Autodesk Inventor part; units mm, degrees
(part 2 of 2)
  spline S89 degree 3 poles (1.5423, -31.1895) (1.525, -31.1709) (1.4965, -31.143) (1.4607, -31.1053) (1.4308, -31.0761) (1.3995, -31.0504) (1.3711, -31.0116) (1.3289, -30.9799) (1.2928, -30.9315) (1.2505, -30.9007) (1.2256, -30.8625) (1.198, -30.8522) (1.1849, -30.8167) (1.168, -30.8425) (1.1747, -30.8641) (1.1731, -30.8896) (1.1714, -30.9248) (1.1764, -30.9669) (1.1759, -31.0225) (1.1727, -31.0799) (1.1753, -31.1417) (1.1771, -31.2039) (1.1741, -31.2647) (1.178, -31.3315) (1.1754, -31.4086) (1.1839, -31.5196) (1.1745, -31.7052) (1.1921, -31.8973) (1.1869, -32.1123) (1.2042, -32.2863) (1.2211, -32.4669) (1.2596, -32.6084) (1.3107, -32.7248) (1.3689, -32.8413) (1.4764, -32.9142) (1.5832, -32.9845) (1.7264, -33.001) (1.8989, -33.0107) (2.1172, -33.0071) (2.3634, -33.008) (2.6188, -33.009) (2.8414, -33.0049) (3.021, -33.0145) (3.147, -32.965) (3.2127, -32.8764) (3.2326, -32.7791) (3.2259, -32.6755) (3.2237, -32.54) (3.2294, -32.3531) (3.2274, -32.1408) (3.2295, -31.893) (3.2271, -31.6251) (3.2278, -31.3115) (3.2293, -31.0183) (3.2271, -30.7799) (3.2306, -30.583) (3.2235, -30.4136) (3.2463, -30.2673) (3.1973, -30.187) (3.166, -30.1309) (3.103, -30.0955) (3.0386, -30.0612) (2.9601, -30.073) (2.877, -30.0634) (2.7737, -30.0639) (2.6629, -30.0682) (2.5435, -30.0645) (2.4271, -30.0598) (2.3642, -30.0653) (2.2866, -30.0561) (2.3231, -30.0866) (2.3537, -30.1027) (2.3857, -30.1444) (2.4192, -30.1889) (2.4599, -30.2542) (2.4978, -30.3242) (2.5079, -30.3954) (2.531, -30.4406) (2.5232, -30.4969) (2.5393, -30.5594) (2.5579, -30.6677) (2.575, -30.8097) (2.5711, -30.9741) (2.5797, -31.1302) (2.5874, -31.2728) (2.58, -31.4046) (2.5875, -31.5255) (2.6027, -31.6432) (2.5734, -31.7683) (2.59, -31.8845) (2.58, -31.9915) (2.5914, -32.0945) (2.5752, -32.2046) (2.5838, -32.3311) (2.5772, -32.4642) (2.5844, -32.5873) (2.5862, -32.686) (2.5777, -32.7699) (2.5862, -32.8154) (2.5728, -32.8827) (2.5522, -32.8428) (2.5299, -32.8211) (2.4929, -32.7958) (2.4669, -32.7597) (2.4326, -32.7361) (2.4064, -32.7076) (2.3753, -32.6805) (2.3475, -32.6496) (2.3163, -32.6216) (2.278, -32.5902) (2.241, -32.5379) (2.1844, -32.4937) (2.1417, -32.4408) (2.0971, -32.398) (2.0525, -32.3645) (2.0209, -32.3209) (1.9846, -32.2913) (1.9485, -32.2523) (1.9142, -32.2193) (1.8787, -32.1788) (1.8467, -32.1411) (1.8016, -32.1072) (1.7684, -32.0675) (1.723, -32.0291) (1.6828, -31.984) (1.6372, -31.9322) (1.5828, -31.8839) (1.5289, -31.8255) (1.4793, -31.7809) (1.4402, -31.742) (1.404, -31.7147) (1.3813, -31.6586) (1.3906, -31.5961) (1.3859, -31.5127) (1.383, -31.4312) (1.3904, -31.37) (1.3777, -31.2946) (1.438, -31.3487) (1.4556, -31.3895) (1.502, -31.4233) (1.5317, -31.4575) (1.5733, -31.4877) (1.5975, -31.5313) (1.6422, -31.5628) (1.6696, -31.6065) (1.7072, -31.6387) (1.7424, -31.6701) (1.7691, -31.7071) (1.8115, -31.7333) (1.8439, -31.7668) (1.8879, -31.8131) (1.9321, -31.8595) (1.9919, -31.9083) (2.0296, -31.9505) (2.0756, -32.0014) (2.1275, -32.0517) (2.1924, -32.1161) (2.2393, -32.1725) (2.2909, -32.2076) (2.3009, -32.2368) (2.3275, -32.2565) (2.3371, -32.233) (2.3277, -32.211) (2.3296, -32.1797) (2.3264, -32.1191) (2.324, -31.9699) (2.3296, -31.6728) (2.3328, -31.2678) (2.3082, -30.8815) (2.2811, -30.6221) (2.2452, -30.4786) (2.2139, -30.3874) (2.1709, -30.31) (2.1288, -30.2355) (2.0582, -30.1918) (1.9981, -30.1354) (1.9228, -30.1164) (1.86, -30.0932) (1.7818, -30.0839) (1.7031, -30.0648) (1.6091, -30.0647) (1.5325, -30.0613) (1.4489, -30.0618) (1.2733, -30.0637) (1.0518, -30.061) (0.7618, -30.0612) (0.5648, -30.0623) (0.3839, -30.0834) (0.3326, -30.1673) (0.2783, -30.2266) (0.2949, -30.2944) (0.277, -30.3586) (0.2876, -30.4558) (0.2771, -30.5742) (0.2899, -30.7018) (0.2803, -30.8207) (0.2884, -30.9299) (0.2664, -31.0532) (0.2756, -31.1752) (0.2699, -31.3079) (0.2729, -31.4304) (0.2665, -31.5576) (0.273, -31.6838) (0.2628, -31.8185) (0.2732, -31.9768) (0.2633, -32.1486) (0.2663, -32.3313) (0.2826, -32.4866) (0.2694, -32.6431) (0.275, -32.7606) (0.2877, -32.8635) (0.3306, -32.9345) (0.4067, -32.9774) (0.5101, -33.0018) (0.6141, -32.994) (0.7167, -33.0028) (0.7978, -33.0003) (0.876, -32.9986) (0.9587, -33.0082) (1.0404, -32.9948) (1.1238, -33.0062) (1.1765, -32.9991) (1.2055, -33.008) knots 0 0 0 0 0.003468 0.005439 0.007104 0.009169 0.010945 0.01361 0.016316 0.01908 0.020762 0.022201 0.023332 0.024029 0.025236 0.026466 0.027456 0.030055 0.032225 0.035047 0.037901 0.04066 0.043548 0.046196 0.049786 0.054063 0.061374 0.07511 0.080331 0.090714 0.098946 0.105065 0.110602 0.11639 0.122413 0.128012 0.133614 0.141696 0.151738 0.163348 0.175333 0.186595 0.193786 0.199727 0.204177 0.208239 0.213025 0.218319 0.226749 0.238544 0.247303 0.260584 0.275108 0.290136 0.300597 0.307698 0.31691 0.324166 0.326546 0.3296 0.33273 0.336239 0.339239 0.343233 0.347669 0.353338 0.35828 0.364316 0.367919 0.369623 0.370752 0.372387 0.375037 0.377468 0.380114 0.385513 0.388136 0.389867 0.392271 0.395601 0.398609 0.407302 0.415055 0.421029 0.428641 0.434538 0.439012 0.445186 0.450585 0.456271 0.461021 0.465216 0.470338 0.476105 0.482456 0.48854 0.492838 0.496163 0.499368 0.500865 0.502042 0.503521 0.505691 0.507878 0.509559 0.511315 0.51315 0.515175 0.516985 0.518877 0.521908 0.525642 0.528599 0.531161 0.53407 0.536151 0.538454 0.540425 0.5434 0.544949 0.547785 0.550125 0.552599 0.554817 0.558226 0.560836 0.564232 0.568141 0.571676 0.573323 0.575691 0.577746 0.581215 0.584106 0.589282 0.591694 0.593826 0.595998 0.598671 0.60089 0.603406 0.604911 0.60784 0.610008 0.61224 0.614777 0.616731 0.618675 0.620926 0.623438 0.625015 0.629649 0.632172 0.635539 0.637359 0.641531 0.645414 0.649794 0.651668 0.653476 0.654327 0.654982 0.656131 0.657628 0.659141 0.664473 0.677942 0.699748 0.719713 0.730811 0.735254 0.739899 0.743899 0.747388 0.751337 0.755043 0.758449 0.761723 0.764177 0.769156 0.772731 0.77696 0.779637 0.78414 0.800935 0.809968 0.823451 0.828907 0.832769 0.836469 0.839009 0.841646 0.845448 0.852184 0.857853 0.86287 0.868439 0.87272 0.879862 0.885038 0.890852 0.896577 0.902417 0.908085 0.914984 0.924029 0.931552 0.939919 0.945276 0.95293 0.955988 0.959308 0.96382 0.967488 0.973717 0.977903 0.981537 0.984789 0.988579 0.992845 0.995948 1 1 1 1 construction
  spline S90 degree 3 poles (2.1147, -31.6416) (2.121, -31.666) (2.1095, -31.6932) (2.1202, -31.731) (2.1024, -31.745) (2.0842, -31.7249) (2.0686, -31.6977) (2.0354, -31.6752) (2.0032, -31.6459) (1.9804, -31.6124) (1.9391, -31.5932) (1.9188, -31.5561) (1.8864, -31.5362) (1.8629, -31.5076) (1.8326, -31.4874) (1.809, -31.447) (1.7749, -31.4194) (1.7277, -31.3803) (1.6926, -31.3305) (1.6462, -31.2905) (1.6081, -31.237) (1.5678, -31.2109) (1.5423, -31.1895) knots 0 0 0 0 0.076447 0.103049 0.115682 0.138833 0.174199 0.229459 0.266643 0.321336 0.361809 0.413983 0.456573 0.486742 0.537524 0.575982 0.641204 0.683051 0.78126 0.843069 0.887588 1 1 1 1 construction
  spline S91 degree 3 poles (1.4623, -30.7315) (1.48, -30.7488) (1.5089, -30.7779) (1.5489, -30.8151) (1.5849, -30.8475) (1.6231, -30.8898) (1.6648, -30.9378) (1.7216, -30.9789) (1.7704, -31.0427) (1.8377, -31.0945) (1.8974, -31.1663) (1.9601, -31.2223) (2.0103, -31.2825) (2.0603, -31.3228) (2.0866, -31.3592) (2.1185, -31.3779) (2.1181, -31.4052) (2.1167, -31.4343) (2.1166, -31.4681) (2.1172, -31.5052) (2.1148, -31.5405) (2.1174, -31.5865) (2.115, -31.6195) (2.1147, -31.6416) knots 0 0 0 0 0.062919 0.104006 0.138611 0.185675 0.248527 0.299493 0.362064 0.450474 0.51321 0.59841 0.663082 0.71174 0.759645 0.777831 0.798589 0.821857 0.854276 0.88334 0.916281 0.943791 1 1 1 1 construction
  line L154 (1.4565, -30.7258) -> (1.4623, -30.7315) construction
  spline S92 degree 3 poles (0.9332, -31.4106) (0.9321, -31.3788) (0.9319, -31.3215) (0.9336, -31.2374) (0.9332, -31.1718) (0.9332, -31.1127) (0.9332, -31.0584) (0.9332, -30.9987) (0.9332, -30.9291) (0.9332, -30.8483) (0.9334, -30.7383) (0.9319, -30.6109) (0.9383, -30.4591) (0.914, -30.3231) (0.9378, -30.2456) (0.9306, -30.2041) (0.9629, -30.2155) (0.9744, -30.2345) (0.9964, -30.2549) (1.0144, -30.2759) (1.0412, -30.297) (1.0642, -30.3274) (1.0912, -30.3569) (1.1173, -30.3827) (1.1375, -30.4029) (1.155, -30.4189) (1.1711, -30.4353) (1.1908, -30.4565) (1.2135, -30.4797) (1.2361, -30.5075) (1.2672, -30.5342) (1.2967, -30.5628) (1.3286, -30.5942) (1.3566, -30.6256) (1.3863, -30.6545) (1.4209, -30.6857) (1.4401, -30.7119) (1.4565, -30.7258) knots 0 0 0 0 0.049219 0.088614 0.130016 0.150735 0.180001 0.213961 0.243067 0.287668 0.338814 0.41337 0.484025 0.576155 0.613926 0.619116 0.629409 0.647447 0.659131 0.674335 0.690575 0.711385 0.732994 0.752394 0.768165 0.777127 0.789028 0.803775 0.821801 0.839329 0.859042 0.885071 0.902859 0.928183 0.95011 0.967011 1 1 1 1 construction
  spline S93 degree 3 poles (1.0224, -32.7673) (1.002, -32.7304) (0.9862, -32.6524) (0.9637, -32.5479) (0.9531, -32.4569) (0.9427, -32.3691) (0.9375, -32.2839) (0.9374, -32.2002) (0.9322, -32.1338) (0.9352, -32.0785) (0.9363, -32.0347) (0.9355, -31.989) (0.9364, -31.9319) (0.9326, -31.8657) (0.9332, -31.7737) (0.9309, -31.6798) (0.9369, -31.5673) (0.922, -31.486) (0.941, -31.4257) (0.9332, -31.4106) knots 0 0 0 0 0.090996 0.174071 0.234828 0.291917 0.3681 0.422099 0.475601 0.514074 0.543605 0.57175 0.614472 0.668944 0.717247 0.816246 0.875574 0.962863 1 1 1 1 construction
  line L155 (4.5438, -2.5813) -> (4.8514, -3.4319) construction
  line L156 (4.6738, -2.5806) -> (4.5438, -2.5813) construction
  spline S94 degree 3 poles (5.9474, -3.4189) (5.9074, -3.4171) (5.8292, -3.4137) (5.715, -3.3994) (5.6069, -3.3792) (5.505, -3.3507) (5.4098, -3.3145) (5.3204, -3.2716) (5.2375, -3.2208) (5.1361, -3.1432) (5.0196, -3.0354) (4.8905, -2.8956) (4.7738, -2.7442) (4.7072, -2.6353) (4.6738, -2.5806) knots 0 0 0 0 0.074854 0.14622 0.21484 0.280346 0.343643 0.405079 0.465383 0.524907 0.643546 0.761548 0.88017 1 1 1 1 construction
  spline S95 degree 3 poles (6.8411, -2.6971) (6.8401, -2.7214) (6.838, -2.7695) (6.8252, -2.84) (6.8049, -2.9075) (6.7777, -2.9724) (6.7435, -3.0346) (6.7016, -3.0938) (6.652, -3.1499) (6.5959, -3.2031) (6.5341, -3.2526) (6.4653, -3.2947) (6.392, -3.3318) (6.3129, -3.3612) (6.2292, -3.3859) (6.1398, -3.4037) (6.0452, -3.4146) (5.9805, -3.4174) (5.9474, -3.4189) knots 0 0 0 0 0.057153 0.11287 0.167856 0.222626 0.277804 0.33431 0.392809 0.453506 0.515764 0.578457 0.642821 0.708485 0.776374 0.847843 0.922215 1 1 1 1 construction
  spline S96 degree 3 poles (5.8268, -1.8734) (5.8878, -1.8825) (6.0083, -1.9005) (6.184, -1.9458) (6.3513, -2.0078) (6.4854, -2.0689) (6.5845, -2.1295) (6.6489, -2.1855) (6.7053, -2.2488) (6.7513, -2.3222) (6.788, -2.4039) (6.8158, -2.494) (6.8336, -2.5927) (6.8386, -2.6614) (6.8411, -2.6971) knots 0 0 0 0 0.127555 0.252046 0.374774 0.496524 0.55651 0.614517 0.672476 0.731397 0.792839 0.857445 0.92603 1 1 1 1 construction
  spline S97 degree 3 poles (4.7368, -1.5247) (4.7649, -1.5454) (4.8233, -1.5887) (4.924, -1.6438) (5.0389, -1.6939) (5.168, -1.7405) (5.3121, -1.7805) (5.4704, -1.8176) (5.6437, -1.8482) (5.7643, -1.8648) (5.8268, -1.8734) knots 0 0 0 0 0.09028 0.18847 0.296589 0.415058 0.54404 0.684309 0.836526 1 1 1 1 construction
  spline S98 degree 3 poles (4.4449, -0.9818) (4.4457, -1.0061) (4.4472, -1.0546) (4.4607, -1.1266) (4.4842, -1.1967) (4.5163, -1.2655) (4.5575, -1.3333) (4.6087, -1.3991) (4.6684, -1.4639) (4.7136, -1.504) (4.7368, -1.5247) knots 0 0 0 0 0.114459 0.228445 0.343049 0.461854 0.585414 0.715802 0.853656 1 1 1 1 construction
  spline S99 degree 3 poles (5.6957, 0.0416) (5.6499, 0.0402) (5.5604, 0.0375) (5.4297, 0.0217) (5.3058, -0.0013) (5.189, -0.0341) (5.0791, -0.0747) (4.9764, -0.1245) (4.8802, -0.1817) (4.7924, -0.2486) (4.7129, -0.3216) (4.6428, -0.4003) (4.5838, -0.4849) (4.5339, -0.5737) (4.4955, -0.6684) (4.4681, -0.7682) (4.4493, -0.8732) (4.4464, -0.9452) (4.4449, -0.9818) knots 0 0 0 0 0.076155 0.148882 0.218511 0.285539 0.350342 0.413066 0.47494 0.536109 0.596202 0.65418 0.710996 0.767236 0.823246 0.880299 0.939171 1 1 1 1 construction
  spline S100 degree 3 poles (6.7309, -0.212) (6.6805, -0.1912) (6.5822, -0.1508) (6.4358, -0.0996) (6.2965, -0.0542) (6.1632, -0.0193) (6.0371, 0.009) (5.9174, 0.0285) (5.8044, 0.0404) (5.7311, 0.0412) (5.6957, 0.0416) knots 0 0 0 0 0.152522 0.297283 0.433646 0.562068 0.68253 0.795182 0.90106 1 1 1 1 construction
  line L157 (6.8853, -0.0736) -> (6.7309, -0.212) construction
  line L158 (6.93, -0.0736) -> (6.8853, -0.0736) construction
  line L159 (7.2938, -0.9097) -> (6.93, -0.0736) construction
  line L160 (7.1594, -0.9097) -> (7.2938, -0.9097) construction
  spline S101 degree 3 poles (5.6957, -0.086) (5.7337, -0.0876) (5.8088, -0.0907) (5.9199, -0.1039) (6.0277, -0.1249) (6.1329, -0.1528) (6.2354, -0.1873) (6.335, -0.2288) (6.431, -0.2787) (6.555, -0.3534) (6.7023, -0.4584) (6.8673, -0.597) (7.0223, -0.7455) (7.1137, -0.8549) (7.1594, -0.9097) knots 0 0 0 0 0.065598 0.129949 0.193003 0.25539 0.317782 0.379718 0.4417 0.504578 0.629795 0.753698 0.87684 1 1 1 1 construction
  spline S102 degree 3 poles (4.698, -0.8708) (4.6997, -0.844) (4.7031, -0.7907) (4.7186, -0.7127) (4.7431, -0.6381) (4.7759, -0.5669) (4.8171, -0.4992) (4.8669, -0.4351) (4.9247, -0.3737) (4.9911, -0.3169) (5.0633, -0.2645) (5.1407, -0.2183) (5.2227, -0.1799) (5.3086, -0.1466) (5.3993, -0.1214) (5.4944, -0.1028) (5.5935, -0.0899) (5.6613, -0.0873) (5.6957, -0.086) knots 0 0 0 0 0.057575 0.114017 0.169688 0.225224 0.281366 0.338833 0.398651 0.461406 0.525502 0.589362 0.653951 0.719063 0.786377 0.854942 0.926213 1 1 1 1 construction
  spline S103 degree 3 poles (5.8268, -1.6072) (5.7713, -1.5978) (5.6645, -1.5798) (5.5121, -1.5484) (5.3744, -1.5128) (5.252, -1.4722) (5.1433, -1.4303) (5.0499, -1.3829) (4.9705, -1.3328) (4.906, -1.2778) (4.8535, -1.2215) (4.8083, -1.1676) (4.7701, -1.1154) (4.7402, -1.064) (4.7173, -1.0141) (4.7036, -0.9649) (4.6957, -0.9173) (4.6972, -0.8861) (4.698, -0.8708) knots 0 0 0 0 0.115586 0.222212 0.319328 0.40724 0.486877 0.558164 0.621984 0.679204 0.731552 0.779719 0.823562 0.864164 0.901543 0.93608 0.968686 1 1 1 1 construction
  spline S104 degree 3 poles (6.8855, -2.0142) (6.8624, -1.99) (6.8139, -1.9395) (6.7231, -1.8758) (6.6163, -1.8168) (6.4918, -1.7639) (6.3505, -1.7156) (6.1913, -1.674) (6.0153, -1.6363) (5.8914, -1.6172) (5.8268, -1.6072) knots 0 0 0 0 0.086611 0.181603 0.286687 0.403128 0.532618 0.674322 0.830229 1 1 1 1 construction
  spline S105 degree 3 poles (7.0942, -2.6146) (7.0935, -2.5866) (7.0922, -2.5314) (7.0821, -2.4498) (7.0664, -2.3706) (7.0435, -2.2939) (7.0131, -2.2203) (6.978, -2.1485) (6.9355, -2.0793) (6.9023, -2.0361) (6.8855, -2.0142) knots 0 0 0 0 0.12951 0.255524 0.379894 0.502709 0.62504 0.747953 0.872309 1 1 1 1 construction
  spline S106 degree 3 poles (5.9474, -3.5465) (5.9863, -3.5455) (6.0627, -3.5436) (6.1747, -3.5295) (6.2825, -3.5103) (6.3853, -3.4811) (6.4843, -3.4464) (6.5779, -3.4021) (6.6676, -3.3515) (6.7514, -3.2927) (6.8291, -3.2285) (6.8968, -3.1571) (6.9549, -3.0804) (7.0031, -2.998) (7.0414, -2.91) (7.0699, -2.8166) (7.0881, -2.7174) (7.0922, -2.6493) (7.0942, -2.6146) knots 0 0 0 0 0.070907 0.139272 0.20577 0.270532 0.334158 0.396982 0.459121 0.521824 0.583484 0.642842 0.700953 0.758596 0.816572 0.875666 0.936543 1 1 1 1 construction
  spline S107 degree 3 poles (5.0541, -3.3226) (5.0971, -3.3406) (5.1806, -3.3756) (5.3044, -3.4226) (5.4234, -3.4613) (5.5377, -3.4929) (5.6469, -3.5171) (5.7514, -3.5349) (5.8511, -3.5449) (5.916, -3.546) (5.9474, -3.5465) knots 0 0 0 0 0.150739 0.292952 0.428208 0.555369 0.676375 0.790082 0.898264 1 1 1 1 construction
  line L161 (4.9007, -3.4319) -> (5.0541, -3.3226) construction
  line L162 (4.8514, -3.4319) -> (4.9007, -3.4319) construction
  spline S108 degree 3 poles (0.1809, -1.7481) (0.1837, -1.8108) (0.1893, -1.9339) (0.2162, -2.1141) (0.2571, -2.2863) (0.3123, -2.4505) (0.3836, -2.6063) (0.4702, -2.7535) (0.57, -2.8939) (0.6853, -3.0234) (0.8109, -3.1423) (0.9473, -3.2462) (1.0919, -3.3358) (1.2462, -3.4084) (1.4086, -3.4672) (1.5797, -3.51) (1.7597, -3.5373) (1.8827, -3.5434) (1.9454, -3.5465) knots 0 0 0 0 0.067074 0.131798 0.194588 0.256201 0.316833 0.377559 0.438695 0.500706 0.562802 0.62348 0.683867 0.744364 0.805604 0.86833 0.932847 1 1 1 1 construction
  line L163 (0.1809, -1.7479) -> (0.1809, -1.7481) construction
  spline S109 degree 3 poles (1.9454, 0.0416) (1.8843, 0.0394) (1.7642, 0.0352) (1.5883, 0.0104) (1.4202, -0.0283) (1.26, -0.0819) (1.1072, -0.1499) (0.9627, -0.2338) (0.8254, -0.3311) (0.6973, -0.4427) (0.5801, -0.567) (0.4772, -0.7034) (0.3891, -0.8507) (0.317, -1.0093) (0.2592, -1.1785) (0.2173, -1.3588) (0.1899, -1.5498) (0.1839, -1.6808) (0.1809, -1.7479) knots 0 0 0 0 0.065198 0.128186 0.189205 0.249021 0.308191 0.367412 0.427014 0.487496 0.548386 0.608955 0.669563 0.731141 0.794468 0.86009 0.928344 1 1 1 1 construction
  spline S110 degree 3 poles (3.7696, -1.7479) (3.7669, -1.681) (3.7617, -1.5501) (3.733, -1.3598) (3.6916, -1.1798) (3.6326, -1.0112) (3.5602, -0.8526) (3.4705, -0.7055) (3.3662, -0.5688) (3.2466, -0.4442) (3.1153, -0.3326) (2.9748, -0.2338) (2.8244, -0.1513) (2.666, -0.082) (2.4979, -0.0292) (2.3218, 0.0107) (2.1365, 0.0352) (2.01, 0.0394) (1.9454, 0.0416) knots 0 0 0 0 0.070085 0.137121 0.201303 0.263318 0.323867 0.383612 0.443363 0.503636 0.564083 0.62372 0.683211 0.743386 0.804636 0.86742 0.932372 1 1 1 1 construction
  spline S111 degree 3 poles (1.9454, -3.5465) (2.01, -3.5437) (2.1367, -3.5382) (2.3219, -3.5106) (2.4984, -3.4685) (2.6659, -3.4107) (2.8252, -3.3386) (2.9747, -3.2498) (3.1157, -3.1466) (3.2466, -3.0293) (3.3657, -2.9001) (3.47, -2.7608) (3.5597, -2.6132) (3.6322, -2.4561) (3.6912, -2.2913) (3.7327, -2.1176) (3.7617, -1.9358) (3.7669, -1.8114) (3.7696, -1.7479) knots 0 0 0 0 0.067917 0.133241 0.196476 0.25841 0.3193 0.379974 0.44082 0.502768 0.564502 0.625247 0.68542 0.74575 0.806846 0.869137 0.933296 1 1 1 1 construction
  line L164 (33.0113, 67.16) -> (-33.0113, 67.16)
  line L165 (-33.0113, 67.16) -> (-33.0113, -67.16)
  line L166 (-33.0113, -67.16) -> (33.0113, -67.16)
  line L167 (33.0113, -67.16) -> (33.0113, 67.16)
  line L168 (40.0113, -74.16) -> (-40.0113, -74.16)
  line L169 (-40.0113, -74.16) -> (-40.0113, 74.16)
  line L170 (-40.0113, 74.16) -> (40.0113, 74.16)
  line L171 (40.0113, 74.16) -> (40.0113, -74.16)
  point P0 (43.5, 39.6821)
  dimension "d0" = 7
  constraints: 16 end point, 4 parallel, 2 perpendicular, 1 horizontal, 3 other
  measures "d0" distance between parallel lines of L166 L168
extrude "Extrusion1" add sketch "Skizze2" along normal blind 2 contours L167 L166 L165 L164 | L168 L169 L170 L171
sketch "Skizze3" plane through (43.5, -39.6821, 19.9558) normal (0, 0, 1) x (1, 0, 0)
  spline S0 degree 3 poles (-35.2897, 69.1115) (-35.2146, 69.1993) (-35.1356, 69.2831) (-35.0534, 69.3629) (-34.983, 69.4312) (-34.9101, 69.4968) (-34.8344, 69.5599) (-34.7663, 69.6167) (-34.6957, 69.6717) (-34.6241, 69.7237) (-34.595, 69.7449) (-34.5657, 69.7656) (-34.5361, 69.7859) (-34.4983, 69.8119) (-34.4602, 69.8372) (-34.4216, 69.8618) (-34.3188, 69.9275) (-34.2133, 69.9887) (-34.1052, 70.0449) (-34.0795, 70.0584) (-34.0536, 70.0715) (-34.0276, 70.0843) (-33.9037, 70.1457) (-33.7765, 70.2008) (-33.6489, 70.2488) knots 0 0 0 0 0.170045 0.170045 0.170045 0.31563 0.31563 0.31563 0.446712 0.446712 0.446712 0.5 0.5 0.5 0.568149 0.568149 0.568149 0.75 0.75 0.75 0.793341 0.793341 0.793341 1 1 1 1
  arc A0 (-35.4977, 68.8443) -> (-36.045, 67.1168) centre (-33.045, 67.1168) ccw
  spline S1 degree 3 poles (33.6489, 70.2488) (33.7763, 70.2009) (33.9028, 70.1461) (34.0267, 70.0848) (34.0529, 70.0718) (34.079, 70.0586) (34.105, 70.0451) (34.2132, 69.9887) (34.3191, 69.9274) (34.4216, 69.8618) (34.4601, 69.8372) (34.4982, 69.812) (34.536, 69.7861) (34.6379, 69.7162) (34.7366, 69.6413) (34.8326, 69.5614) (34.9087, 69.498) (34.9823, 69.4319) (35.053, 69.3633) (35.1355, 69.2832) (35.2145, 69.1993) (35.2897, 69.1115) knots 0 0 0 0 0.206366 0.206366 0.206366 0.25 0.25 0.25 0.431731 0.431731 0.431731 0.5 0.5 0.5 0.683994 0.683994 0.683994 0.829787 0.829787 0.829787 1 1 1 1
  arc A1 (36.045, 67.1168) -> (35.4977, 68.8443) centre (33.045, 67.1168) ccw
  spline S2 degree 3 poles (33.6489, -70.2488) (34.3839, -69.9724) (35.0488, -69.4815) (35.4977, -68.8443) knots 0.181743 0.181743 0.181743 0.181743 0.689724 0.689724 0.689724 0.689724
  arc A2 (35.4977, -68.8443) -> (36.045, -67.1168) centre (33.045, -67.1168) ccw
  spline S3 degree 3 poles (-33.6489, -70.2488) (-33.7763, -70.2009) (-33.9028, -70.1461) (-34.0267, -70.0848) (-34.0529, -70.0718) (-34.079, -70.0586) (-34.105, -70.0451) (-34.2132, -69.9887) (-34.3191, -69.9274) (-34.4216, -69.8618) (-34.4601, -69.8372) (-34.4982, -69.812) (-34.536, -69.7861) (-34.6379, -69.7162) (-34.7366, -69.6413) (-34.8326, -69.5614) (-34.9087, -69.498) (-34.9823, -69.4319) (-35.053, -69.3633) (-35.1355, -69.2832) (-35.2145, -69.1993) (-35.2897, -69.1115) knots 0 0 0 0 0.206366 0.206366 0.206366 0.25 0.25 0.25 0.431731 0.431731 0.431731 0.5 0.5 0.5 0.683994 0.683994 0.683994 0.829787 0.829787 0.829787 1 1 1 1
  arc A3 (-36.045, -67.1168) -> (-35.4977, -68.8443) centre (-33.045, -67.1168) ccw
  line L0 (-40.0113, -74.16) -> (40.0113, -74.16)
  line L1 (40.0113, -74.16) -> (40.0113, 74.16)
  line L2 (40.0113, 74.16) -> (-40.0113, 74.16)
  line L3 (-40.0113, 74.16) -> (-40.0113, -74.16)
  line L4 (-37.5, -72) -> (37.5, -72)
  line L5 (37.5, -72) -> (37.5, 72)
  line L6 (37.5, 72) -> (-37.5, 72)
  line L7 (-37.5, 72) -> (-37.5, -72)
  line L8 (-37.5, -72) -> (37.5, 72) construction
  line L9 (37.5, -72) -> (-37.5, 72) construction
  point P0 (-43.5, 39.6821)
  point P1 (0, 0)
  dimension "d3" = 75
  dimension "d4" = 144
  constraints: 12 end point, 2 midpoint, 2 parallel, 1 horizontal, 1 perpendicular
  measures "d3" distance of L6.end L5.end
  measures "d4" distance of L5.end L4.end
extrude "Extrusion2" add sketch "Skizze3" along normal blind 6
sketch "Skizze4" plane through (43.5, -39.6821, 25.9558) normal (0, 0, 1) x (1, 0, 0)
  spline S0 degree 3 poles (35.8524, -47.4044) (35.8524, -47.6205) (35.8698, -47.8496) (35.9265, -48.2694) (35.9641, -48.4605) (36.0215, -48.7638) (36.0449, -48.8959) (36.045, -48.9832) (36.045, -48.9834) (36.045, -48.9836) knots 0 0 0 0 0.332822 0.332822 0.665644 0.665644 0.999252 0.999252 1 1 1 1
  line L0 (35.545, -49.1121) -> (35.545, -47.4044)
  line L1 (35.545, -27.4535) -> (35.545, -25.7458)
  line L2 (34.045, -10.4041) -> (34.045, -8.0936)
  line L3 (34.045, 7.8983) -> (34.045, 10.2089)
  line L4 (-36.345, -5.5736) -> (-36.345, -10.4264)
  line L5 (-36.045, -55.0588) -> (-36.045, -18.7142)
  line L6 (-36.045, -1.4127) -> (-36.045, -1.6995)
  line L7 (-36.045, 19.0928) -> (-36.045, 18.806)
  line L8 (-37.5, -72) -> (-37.5, 72)
  line L9 (-37.5, 72) -> (37.5, 72)
  line L10 (37.5, 72) -> (37.5, -72)
  line L11 (37.5, -72) -> (-37.5, -72)
  line L12 (-40.0113, -74.16) -> (40.0113, -74.16)
  line L13 (40.0113, -74.16) -> (40.0113, 74.16)
  line L14 (40.0113, 74.16) -> (-40.0113, 74.16)
  line L15 (-40.0113, 74.16) -> (-40.0113, -74.16)
  line L16 (-37.5, -72) -> (-37.5, 72)
  line L17 (-40.0113, 74.16) -> (-40.0113, -74.16)
  line L18 (-37.5, -56.1519) -> (-40.0113, -56.1519)
  line L19 (-40.0113, -56.1519) -> (-40.0113, 23.8455)
  line L20 (-40.0113, 23.8455) -> (-37.5, 23.8455)
  line L21 (-37.5, 23.8455) -> (-37.5, -56.1519)
  line L22 (37.5, -72) -> (37.5, 72)
  line L23 (40.0113, -74.16) -> (40.0113, 74.16)
  line L24 (37.5, -54.5381) -> (40.0113, -54.5381)
  line L25 (40.0113, -54.5381) -> (40.0113, 24.4085)
  line L26 (40.0113, 24.4085) -> (37.5, 24.4085)
  line L27 (37.5, 24.4085) -> (37.5, -54.5381)
  point P0 (-43.5, 39.6821)
  constraints: 16 end point, 4 parallel, 4 point on line, 2 horizontal, 2 perpendicular
extrude "Extrusion3" cut sketch "Skizze4" against normal up to surface (6 mm away) contours L18 L15 L20 L8 | L10 L26 L13 L24
sketch "Skizze5" plane through (43.5, -39.6821, 17.9558) normal (0, 0, -1) x (-1, 0, 0)
  circle A0 centre (20, -59.8179) radius 9.5 projected
  point P0 (43.5, 39.6821)
extrude "Extrusion4" cut sketch "Skizze5" against normal blind 4
sketch "Skizze6" plane through (43.5, -39.6821, 17.9558) normal (0, 0, -1) x (-1, 0, 0)
  circle A0 centre (20, -59.8179) radius 9.5 projected
  line L0 (-40.0113, -74.16) -> (40.0113, -74.16) construction
  line L1 (40.0113, -74.16) -> (40.0113, 74.16) construction
  line L2 (40.0113, 74.16) -> (-40.0113, 74.16) construction
  line L3 (-40.0113, 74.16) -> (-40.0113, -74.16) construction
  line L4 (-35.0113, -69.16) -> (35.0113, -69.16) construction
  line L5 (35.0113, -69.16) -> (35.0113, 69.16) construction
  line L6 (35.0113, 69.16) -> (-35.0113, 69.16) construction
  line L7 (-35.0113, 69.16) -> (-35.0113, -69.16) construction
  circle A1 centre (35.0113, 35.0572) radius 2.5
  circle A2 centre (35.0113, -69.16) radius 2.5
  circle A3 centre (-5, -69.16) radius 2.5
  circle A4 centre (-5, 35.0572) radius 2.5
  point P0 (43.5, 39.6821)
  dimension "d11" = 5
  dimension "d12" = 5
  dimension "d13" = 5
  dimension "d14" = 5
  dimension "d15" = 9.6669
  dimension "d16" = 48.72
  dimension "d17" = 119.1589
  dimension "d18" = 118.1287
  constraints: 8 end point, 4 centre point, 2 point on line, 1 coincident, 1 equal radius, 3 other
  measures "d11" distance between parallel lines of L3 L7
  measures "d12" diameter of A1
  measures "d13" diameter of A2
  measures "d14" diameter of A3
  measures "d15" distance of point (43.5, 39.682) A1.centre
  measures "d16" distance of point (43.5, 39.682) A4.centre
  measures "d17" distance of point (43.5, 39.682) A3.centre
  measures "d18" distance of L0.end A4.centre
extrude "Extrusion5" cut sketch "Skizze6" against normal through all contours A1 | A2 | A3 | A4
fillet "Rundung1" radius 3 15 edges at (82.2556, -94.2202, 25.9558) (82.2556, -94.2202, 19.9558) (4.7444, -95.8341, 25.9558) (4.7444, -95.8341, 19.9558) (82.2556, -15.2736, 25.9558) (82.2556, -15.2736, 19.9558) (4.7444, -15.8366, 19.9558) (4.7444, -15.8366, 25.9558) (83.5113, 34.4779, 21.9558) (3.4887, 34.4779, 21.9558) (6, 32.3179, 22.9558) (81, 32.3179, 22.9558) (83.5113, -113.8421, 21.9558) (3.4887, -113.8421, 21.9558) (81, -111.6821, 22.9558)
